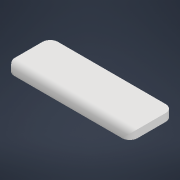
# Autodesk Inventor part: Подставка1
Saved by Autodesk Inventor 2022 (Build 260153000, 153)
## iProperties
Created: 2021-11-11
Part Number: Подставка1
Material: Типовые
Document SubType Name: Modeling
Designer: olegs
Density: 1 g/cm^3
Appearance: По умолчанию
Author: olegs
Autodesk Inventor part; units mm, degrees
ref_plane "YZ Plane" through (0, 0, 0) normal (1, 0, 0) x (0, 1, 0)
ref_plane "XZ Plane" through (0, 0, 0) normal (0, 1, 0) x (-1, 0, 0)
ref_plane "XY Plane" through (0, 0, 0) normal (0, 0, 1) x (1, 0, 0)
sketch "Эскиз1" plane through (0, 0, 0) normal (0, 1, 0) x (-1, 0, 0)
  line L0 (35, -85) -> (-445, -85)
  line L1 (-445, -85) -> (-445, 85)
  line L2 (-445, 85) -> (35, 85)
  line L3 (35, 85) -> (35, -85)
  point P0 (0, 0)
  point P1 (35, 0)
  dimension "d0" = 480
  dimension "d1" = 170
  dimension "d2" = 35
  constraints: 8 end point, 2 parallel, 1 horizontal, 1 horizontal alignment, 1 midpoint, 1 perpendicular
  measures "d0" distance of L1.end L2.end
  measures "d1" distance of L0.end L1.end
  measures "d2" distance from line of point (0, 0) L3
extrude "Выдавливание1" add sketch "Эскиз1" along normal mid plane 30
fillet "Сопряжение1" radius 30 5 edges at (445, 0, 85) (-35, 0, 85) (445, 0, -85) (-35, 0, -85) (205, 15, 85)
